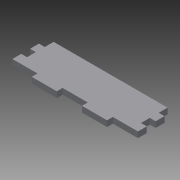
# Autodesk Inventor part: cajon lat
Saved by Autodesk Inventor 2015 (Build 190159000, 159)
## iProperties
Created: 2016-01-26
Part Number: cajon lat
Material: Generic
Document SubType Name: Modeling
Designer: iberopuebla
Density: 1 g/cm^3
Appearance: Default
Author: iberopuebla
Autodesk Inventor part; units mm, degrees
ref_plane "YZ Plane" through (0, 0, 0) normal (1, 0, 0) x (0, 1, 0)
ref_plane "XZ Plane" through (0, 0, 0) normal (0, 1, 0) x (-1, 0, 0)
ref_plane "XY Plane" through (0, 0, 0) normal (0, 0, 1) x (1, 0, 0)
sketch "Sketch1" plane through (0, 0, 0) normal (0, 0, 1) x (1, 0, 0)
  line L0 (372, 110) -> (18, 110)
  line L1 (78, 0) -> (78, -18)
  line L2 (156, 0) -> (156, -18)
  line L3 (234, 0) -> (234, -18)
  line L4 (312, 0) -> (312, -18)
  line L5 (78, -18) -> (156, -18)
  line L6 (234, -18) -> (312, -18)
  line L7 (156, 0) -> (234, 0)
  line L8 (18, 27.5) -> (0, 27.5)
  line L9 (18, 55) -> (0, 55)
  line L10 (18, 55) -> (0, 55)
  line L11 (18, 82.5) -> (0, 82.5)
  line L12 (390, 82.5) -> (372, 82.5)
  line L13 (390, 55) -> (372, 55)
  line L14 (390, 27.5) -> (372, 27.5)
  line L15 (0, 0) -> (0, 27.5)
  line L16 (0, 55) -> (0, 82.5)
  line L17 (390, 0) -> (390, 27.5)
  line L18 (390, 55) -> (390, 82.5)
  line L19 (372, 27.5) -> (372, 55)
  line L20 (372, 82.5) -> (372, 110)
  line L21 (18, 110) -> (18, 82.5)
  line L22 (18, 55) -> (18, 27.5)
  line L23 (312, 0) -> (390, 0)
  line L24 (0, 0) -> (78, 0)
  dimension "d7" = 78
  dimension "d8" = 78
  dimension "d9" = 78
  dimension "d11" = 18
  dimension "d12" = 18
  dimension "d13" = 18
  dimension "d24" = 18
  dimension "d25" = 18
  dimension "d26" = 18
  dimension "d28" = 18
  dimension "d32" = 18
  dimension "d33" = 18
  dimension "d35" = 78
  dimension "d36" = 78
  dimension "d39" = 27.5
  dimension "d40" = 27.5
  dimension "d41" = 27.5
  dimension "d42" = 27.5
  dimension "d48" = 27.5
  dimension "d49" = 27.5
  dimension "d50" = 27.5
  dimension "d51" = 27.5
  dimension "d52" = 110
  constraints: 50 end point, 16 perpendicular, 9 parallel, 5 horizontal, 2 vertical, 1 coincident
  measures "d7" distance between parallel lines of L2 L1
  measures "d8" distance between parallel lines of L3 L2
  measures "d9" distance between parallel lines of L4 L3
  measures "d11" distance of L2.start L2.end
  measures "d12" distance of L3.start L3.end
  measures "d13" distance of L4.start L4.end
  measures "d24" horizontal distance of L17.start L14.end
  measures "d25" distance of L13.start L13.end
  measures "d26" distance of L12.start L12.end
  measures "d28" distance of L9.start L9.end
  measures "d32" distance of L8.start L8.end
  measures "d33" distance of L11.start L11.end
  measures "d35" distance between parallel lines of L15 L1
  measures "d36" distance between parallel lines of L17 L4
  measures "d39" distance of L15.start L8.end
  measures "d40" distance of L9.start L8.start
  measures "d41" distance of L9.end L11.end
  measures "d42" distance of L0.end L11.start
  measures "d48" distance of L17.start L14.start
  measures "d49" distance of L14.end L13.end
  measures "d50" distance of L13.start L12.start
  measures "d51" distance of L12.end L0.start
  measures "d52" distance from line of L0 point (0, 0)
extrude "Extrusion3" add sketch "Sketch1" along normal blind 18
body "Solid3"
